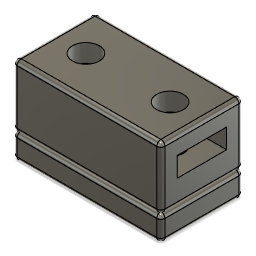
Belt Clip (Autodesk Fusion 360 design; units mm, degrees)
Autodesk Fusion 360 part; units mm, degrees
note: some values were not read from the file. Set by a fixed rule: which face or edge a step refers to.
sketch "Sketch1" plane through (0, 0, 0) normal (0, 1, 0) x (1, 0, 0)
  line L0 (0, 0) -> (18, 0)
  line L1 (18, 0) -> (18, 10)
  line L2 (18, 10) -> (0, 10)
  line L3 (0, 10) -> (0, 0)
  line L4 (0, 5) -> (18, 5) construction
  line L5 (7.3391, 5) -> (5.6071, 8)
  line L6 (5.6071, 8) -> (2.1429, 8)
  line L7 (2.1429, 8) -> (0.4109, 5) construction
  line L8 (0.4109, 5) -> (2.1429, 2) construction
  line L9 (2.1429, 2) -> (5.6071, 2)
  line L10 (5.6071, 2) -> (7.3391, 5)
  line L11 (15.8571, 8) -> (12.3929, 8)
  line L12 (12.3929, 8) -> (10.6609, 5)
  line L13 (10.6609, 5) -> (12.3929, 2)
  line L14 (12.3929, 2) -> (15.8571, 2)
  line L15 (15.8571, 2) -> (17.5891, 5) construction
  line L16 (17.5891, 5) -> (15.8571, 8) construction
  line L17 (2.1429, 8) -> (0, 8)
  line L18 (2.1429, 2) -> (0, 2)
  line L19 (15.8571, 8) -> (18, 8)
  line L20 (15.8571, 2) -> (18, 2)
  circle A0 centre (14.125, 5) radius 1.625
  circle A1 centre (3.875, 5) radius 1.625
  line L21 (7.3391, 5) -> (10.6609, 5) construction
  point P0 (3.875, 5)
  point P1 (14.125, 5)
  dimension "d2" = 3
  dimension "d3" = 3.25
  dimension "d4" = 3.25
  dimension "d5" = 10
  dimension "d6" = 18
  dimension "d8" = 3
  dimension "d9" = 10.25
  constraint horizontal L0
  constraint vertical L1
  constraint horizontal L2
  constraint vertical L3
  constraint coincident L0.start L3.end
  constraint midpoint L3 L4.start
  constraint midpoint L1 L4.end
  constraint coincident L4 P0
  constraint coincident L4 P1
  constraint horizontal L11
  constraint horizontal L6
  constraint coincident L3 L17.end
  constraint perpendicular L3 L17
  constraint coincident L3 L18.end
  constraint perpendicular L3 L18
  constraint coincident L1 L19.end
  constraint perpendicular L1 L19
  constraint coincident L1 L20.end
  constraint perpendicular L1 L20
  constraint coincident P1 A0.centre
  constraint coincident P0 A1.centre
  constraint midpoint L4 L21
  measures "d2" distance of P1 L16
  measures "d3" diameter of A0
  measures "d4" diameter of A1
  measures "d5" distance of L0.start L2.end
  measures "d6" distance of L1.end L2.end
  measures "d8" distance of L8 P0
  measures "d9" distance of P1 P0
extrude "Extrude1" add sketch "Sketch1" along normal blind 7.6 contours L0 L1 L2 L3 L5 L6 L9 L10 L11 L12 L13 L14 L17 L18 L19 L20 | L3 L5 L6 L9 L10 L17 L18 | L1 L11 L12 L13 L14 L19 L20 | A0 | A1 makes body 1
extrude "Extrude2" cut sketch "Sketch1" along normal blind 2.4 from surface at 3 contours L3 L5 L6 L9 L10 L17 L18 | L1 L11 L12 L13 L14 L19 L20 bodies 1
extrude "Extrude3" cut sketch "Sketch1" along normal up to surface (7.6 mm away) contours A0 | A1 bodies 1
extrude "Extrude4" add sketch "Sketch1" against normal blind 3 separate body makes body 2
fillet "Fillet1" radius 0.5 4 edges at (18, 7.6, -5) (18, 0, -5) (0, 0, -5) (0, 7.6, -5) 2 faces at (6, 5.0667, -10) (12, 5.0667, 0) on bodies 1
fillet "Fillet2" radius 0.5 4 faces at (0, -2, -0.6667) (12, -2, -10) (6, -2, 0) (18, -1, -0.6667) on bodies 2
equation "d2 = 5.5 mm / 2 + 0.25 mm"
equation "d8 = ( 5.5 / 2 ) * 1 mm + 0.25 mm"
equation "d9 = d3 + 7 mm"
equation "d10 = 10 mm - 2.4 mm"
